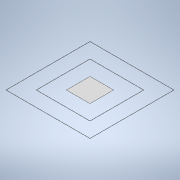
# Autodesk Inventor part: Part1
Saved by Autodesk Inventor 2022 (Build 260153000, 153)
## iProperties
Created: 2022-04-01
Part Number: Part1
Material: Generic
Document SubType Name: Modeling
Designer: torba
Density: 1 g/cm^3
Appearance: Default
Author: torba
Autodesk Inventor part; units mm, degrees
ref_plane "YZ Plane" through (0, 0, 0) normal (1, 0, 0) x (0, 1, 0)
ref_plane "XZ Plane" through (0, 0, 0) normal (0, 1, 0) x (-1, 0, 0)
ref_plane "XY Plane" through (0, 0, 0) normal (0, 0, 1) x (1, 0, 0)
sketch "Sketch1" plane through (0, 0, 0) normal (0, 1, 0) x (-1, 0, 0)
  line L0 (0, 0) -> (300, 0) construction
  line L1 (300, 0) -> (300, -300) construction
  line L2 (300, -300) -> (0, -300) construction
  line L3 (0, -300) -> (0, 0) construction
  line L4 (290, -290) -> (290, -10) construction
  line L5 (290, -10) -> (10, -10) construction
  line L6 (10, -10) -> (10, -290) construction
  line L7 (10, -290) -> (290, -290) construction
  line L8 (290, -10) -> (10, -10)
  line L9 (10, -10) -> (10, -290)
  line L10 (10, -290) -> (290, -290)
  line L11 (290, -290) -> (290, -10)
  line L12 (289.6, -10.4) -> (289.6, -289.6)
  line L13 (289.6, -289.6) -> (10.4, -289.6)
  line L14 (10.4, -289.6) -> (10.4, -10.4)
  line L15 (10.4, -10.4) -> (289.6, -10.4)
  line L16 (239.6, -239.6) -> (239.6, -60.4)
  line L17 (239.6, -60.4) -> (60.4, -60.4)
  line L18 (60.4, -60.4) -> (60.4, -239.6)
  line L19 (60.4, -239.6) -> (239.6, -239.6)
  line L20 (239.2, -60.8) -> (239.2, -239.2)
  line L21 (239.2, -239.2) -> (60.8, -239.2)
  line L22 (60.8, -239.2) -> (60.8, -60.8)
  line L23 (60.8, -60.8) -> (239.2, -60.8)
  line L24 (189.2, -189.2) -> (189.2, -110.8)
  line L25 (189.2, -110.8) -> (110.8, -110.8)
  line L26 (110.8, -110.8) -> (110.8, -189.2)
  line L27 (110.8, -189.2) -> (189.2, -189.2)
  line L28 (188.8, -111.2) -> (188.8, -188.8)
  line L29 (188.8, -188.8) -> (111.2, -188.8)
  line L30 (111.2, -188.8) -> (111.2, -111.2)
  line L31 (111.2, -111.2) -> (188.8, -111.2)
  line L32 (157.5, -157.5) -> (157.5, -142.5)
  line L33 (157.5, -142.5) -> (142.5, -142.5)
  line L34 (142.5, -142.5) -> (142.5, -157.5)
  line L35 (142.5, -157.5) -> (157.5, -157.5)
  dimension "d0" = 300
  dimension "d1" = 300
  dimension "d2" = 10
  dimension "d3" = 0.4
  dimension "d4" = 50
  dimension "d5" = 0.4
  dimension "d6" = 50
  dimension "d7" = 0.4
  dimension "d8" = 15
  constraints: 72 end point, 9 perpendicular, 6 parallel, 2 horizontal, 21 other
  measures "d0" distance of L1.end L2.end
  measures "d1" distance of L0.end L1.end
  measures "d2" distance between parallel lines of L1 L4
  measures "d3" distance between parallel lines of L4 L12
  measures "d4" distance between parallel lines of L12 L16
  measures "d5" distance between parallel lines of L16 L20
  measures "d6" distance between parallel lines of L20 L24
  measures "d7" distance between parallel lines of L24 L28
  measures "d8" distance between parallel lines of L35 L33
extrude "Extrusion1" add sketch "Sketch1" along normal blind 0.1 contours L11 L10 L9 L8 | L19 L18 L17 L16 | L27 L26 L25 L24 | L28 L29 L30 L31 | L35 L34 L33 L32
body "Solid1"
